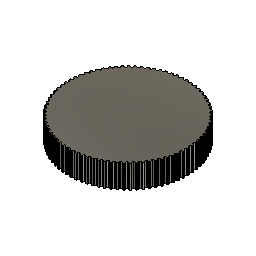
gear_81z (Autodesk Fusion 360 design; units mm, degrees)
Autodesk Fusion 360 part; units mm, degrees
sketch "Sketch1" plane through (0, 0, 0) normal (0, 0, 1) x (1, 0, 0) in component "gt2 pulley"
  circle A0 centre (0, 0) radius 25.7831 construction
  circle A1 centre (0, 0) radius 24.7791 construction
  line L0 (0, 0) -> (0, 25.7831) construction
  line L1 (0, 0) -> (0.9997, 25.7637) construction
  line L2 (0, 0) -> (1.4048, 25.7448) construction
  circle A2 centre (0, 0) radius 25.5291 construction
  arc A3 (0.3959, 25.3927) -> (0.4727, 25.0954) centre (1.391, 25.4912) ccw
  circle A4 centre (0, 0) radius 25.3791 construction
  arc A5 (0.248, 25.5279) -> (0, 25.5291) centre (0, 0) ccw
  arc A6 (0.3959, 25.3927) -> (0.248, 25.5279) centre (0.2466, 25.3779) ccw
  arc A7 (0.4727, 25.0954) -> (0.9608, 24.7605) centre (0.9823, 25.315) ccw
  arc A8 (0, 25.5291) -> (-0.248, 25.5279) centre (0, 0) ccw
  arc A9 (-0.248, 25.5279) -> (-0.3959, 25.3927) centre (-0.2466, 25.3779) ccw
  arc A10 (-0.4727, 25.0954) -> (-0.3959, 25.3927) centre (-1.391, 25.4912) ccw
  arc A11 (-0.9607, 24.7605) -> (-0.4727, 25.0954) centre (-0.9823, 25.315) ccw
  arc A12 (0.9608, 24.7605) -> (-0.9608, 24.7605) centre (0, 0) ccw
  point P0 (1.391, 25.4912)
  point P1 (0, 25.5291)
  dimension "d18" = 51.5662
  dimension "d19" = 2.222
  dimension "d22" = 1.004
  dimension "d24" = 0.75
  dimension "d26" = 1
  dimension "d27" = 0.15
  dimension "d28" = 0.15
  dimension "d47" = 0.555
  dimension "d52" = 3.812
  constraint coincident A0.centre A1.centre
  constraint coincident A0 L0.end
  constraint vertical L0
  constraint coincident A0 L1.end
  constraint coincident A0 L2.end
  constraint concentric A1 A2
  constraint coincident A1 A7.end
  constraint coincident L1 A7.end
  constraint coincident A2 P0
  constraint coincident L2 P0
  constraint coincident P0 A3.centre
  constraint coincident A2 P1
  constraint coincident L0 P1
  constraint concentric A2 A4
  constraint coincident P1 A5.end
  constraint coincident A4 A6.centre
  constraint coincident A3.start A6.start
  constraint tangent A3 A6
  constraint tangent A3 A7
  constraint symmetric L0 A7.end A12.end
  constraint symmetric L0 A3.start A9.end
  constraint symmetric L0 A3.end A10.start
  constraint symmetric L0 A3 A10
  constraint symmetric L0 A5.start A8.end
  constraint symmetric L0 P1 A5.end
  constraint symmetric L0 A5 A8
  constraint symmetric L0 A6 A9
  constraint symmetric L0 A7 A11
  constraint coincident A1 A11.start
  constraint tangent A1 A7
  constraint coincident L1 A7.centre
  measures "d18" diameter of A0
  measures "d19" angle of L0 L1
  measures "d22" distance of A0 A1
  measures "d24" distance of A1 A2
  measures "d26" radius of A3
  measures "d27" distance of A2 A4
  measures "d28" radius of A6
  measures "d47" radius of A7
extrude "Extrude1" add sketch "Sketch1" along normal blind 10 makes body 1
pattern_circular "C-Pattern1" count 81 over 360 about axis through (0, 0, 1.75) along (0, 0, 1) of bodies 1 makes body 2 at (-1.1742, 24.7513, 3.3333) makes body 3 at (-4.3553, 24.3933, 6.6667) makes body 4 at (-4.9846, 24.2726, 3.3333) makes body 5 at (-8.0723, 23.4274, 6.6667) makes body 6 at (-8.6753, 23.2108, 3.3333) makes body 7 at (-11.7836, 21.798, 6.6667) makes body 8 at (-12.1576, 21.5916, 3.3333) makes body 9 at (-14.8398, 19.844, 6.6667) makes body 10 at (-16.4929, 18.4929, 6.6667) makes body 11 at (-17.7278, 17.3126, 6.6667) makes body 12 at (-18.1695, 16.8485, 3.3333) makes body 13 at (-19.9394, 14.7113, 6.6667) makes body 14 at (-21.0195, 13.1219, 6.6667) makes body 15 at (-22.1673, 11.0732, 6.6667) makes body 16 at (-22.7946, 9.7164, 6.6667) makes body 17 at (-23.1921, 8.7253, 3.3333) makes body 18 at (-24.0222, 6.0775, 6.6667) makes body 19 at (-24.5213, 3.5649, 6.6667) makes body 20 at (-24.5791, 3.1417, 3.3333) makes body 21 at (-24.7487, 1.2275, 3.3333) makes body 22 at (-24.6825, -2.1862, 6.6667) makes body 23 at (-24.4388, -4.0923, 6.6667) makes body 24 at (-24.3647, -4.513, 3.3333) makes body 25 at (-23.513, -7.8194, 6.6667) makes body 26 at (-23.1543, -8.8251, 6.6667) makes body 27 at (-22.3086, -10.7856, 6.6667) makes body 28 at (-21.8233, -11.7367, 3.3333) makes body 29 at (-20.8481, -13.3925, 3.3333) makes body 30 at (-19.7476, -14.9678, 3.3333) makes body 31 at (-18.5284, -16.4531, 3.3333) makes body 32 at (-16.0908, -18.8439, 6.6667) makes body 33 at (-14.5821, -20.0341, 6.6667) makes body 34 at (-14.2346, -20.2825, 3.3333) makes body 35 at (-11.5009, -21.9484, 6.6667) makes body 36 at (-9.5689, -22.857, 6.6667) makes body 37 at (-7.7689, -23.5297, 6.6667) makes body 38 at (-5.9221, -24.061, 6.6667) makes body 39 at (-4.6705, -24.335, 6.6667) makes body 40 at (-2.3458, -24.6678, 6.6667) makes body 41 at (-1.7072, -24.7202, 3.3333) makes body 42 at (1.7071, -24.7202, 6.6667) makes body 43 at (2.133, -24.6871, 3.3333) makes body 44 at (5.5064, -24.1596, 6.6667) makes body 45 at (6.7478, -23.8426, 6.6667) makes body 46 at (8.3745, -23.3211, 6.6667) makes body 47 at (10.9295, -22.2385, 6.6667) makes body 48 at (11.3113, -22.0467, 3.3333) makes body 49 at (12.9857, -21.1039, 3.3333) makes body 50 at (14.5821, -20.0342, 3.3333) makes body 51 at (16.0907, -18.8439, 3.3333) makes body 52 at (18.5283, -16.4532, 6.6667) makes body 53 at (18.8092, -16.1313, 3.3333) makes body 54 at (20.4949, -13.9271, 6.6667) makes body 55 at (21.5125, -12.297, 6.6667) makes body 56 at (22.4007, -10.593, 6.6667) makes body 57 at (23.3747, -8.2237, 6.6667) makes body 58 at (23.9416, -6.3876, 6.6667) makes body 59 at (24.3646, -4.5131, 6.6667) makes body 60 at (24.4388, -4.0924, 3.3333) makes body 61 at (24.6825, -2.1862, 3.3333) makes body 62 at (24.7777, -0.267, 3.3333) makes body 63 at (24.7238, 1.6539, 3.3333) makes body 64 at (24.3839, 4.4079, 6.6667) makes body 65 at (23.7985, 6.9018, 6.6667) makes body 66 at (23.676, 7.311, 3.3333) makes body 67 at (23.0382, 9.1238, 3.3333) makes body 68 at (21.5654, 12.2041, 6.6667) makes body 69 at (20.5548, 13.8385, 6.6667) makes body 70 at (19.4206, 15.3897, 6.6667) makes body 71 at (18.1696, 16.8484, 6.6667) makes body 72 at (17.8764, 17.1592, 3.3333) makes body 73 at (15.348, 19.4536, 6.6667) makes body 74 at (14.4956, 20.0968, 6.6667) makes body 75 at (13.4374, 20.8192, 3.3333) makes body 76 at (11.7837, 21.7979, 3.3333) makes body 77 at (10.0591, 22.6455, 3.3333) makes body 78 at (6.8507, 23.8133, 6.6667) makes body 79 at (4.9847, 24.2725, 6.6667) makes body 80 at (4.5655, 24.3549, 3.3333) makes body 81 at (1.1743, 24.7513, 6.6667)
sketch "Sketch2" plane through (0, 0, 10) normal (0, 0, 1) x (-1, 0, 0)
  arc A0 (-11.75, -22.5141) -> (-11.6785, -22.7013) centre (-11.6099, -22.5679) ccw
  arc A1 (-11.6785, -22.7013) -> (-11.2353, -22.9239) centre (0, 0) ccw
  arc A2 (-11.2353, -22.9239) -> (-11.0425, -22.8694) centre (-11.1692, -22.7892) ccw
  arc A3 (-10.8404, -22.6382) -> (-11.0425, -22.8694) centre (-10.1974, -23.404) ccw
  arc A4 (-10.2539, -22.5579) -> (-10.8404, -22.6382) centre (-10.4835, -23.0632) ccw
  arc A5 (-11.9711, -21.6955) -> (-10.2539, -22.5579) centre (0, 0) ccw
  arc A6 (-11.6852, -22.2139) -> (-11.9711, -21.6955) centre (-12.2392, -22.1815) ccw
  arc A7 (-11.75, -22.5141) -> (-11.6852, -22.2139) centre (-12.6835, -22.1555) ccw
  circle A8 centre (0, 0) radius 24.7791
  constraint concentric A1 A8
extrude "Extrude2" add sketch "Sketch2" against normal blind 10 contours A5 A8 bodies 1 2 3 4 5 6 7 8 9 10 11 12 13 14 15 16 17 18 19 20 21 22 23 24 25 26 27 28 29 30 31 32 33 34 35 36 37 38 39 40 41 42 43 44 45 46 47 48 49 50 51 52 53 54 55 56 57 58 59 60 61 62 63 64 65 66 67 68 69 70 71 72 73 74 75 76 77 78 79 80 81
extrude "Extrude4" [suppressed] in component "gt2 pulley"
pattern_circular "C-Pattern7" [suppressed] in component "gt2 pulley"
extrude "Extrude3" [suppressed] in component "gt2 pulley"
pattern_circular "C-Pattern6" [suppressed] in component "gt2 pulley"
extrude "Extrude2'" [suppressed] in component "gt2 pulley"
pattern_circular "C-Pattern5" [suppressed] in component "gt2 pulley"
extrude "Extrude1'" [suppressed] in component "gt2 pulley"
pattern_circular "C-Pattern4" [suppressed] in component "gt2 pulley"
pattern_circular "C-Pattern3" [suppressed] in component "gt2 pulley"
pattern_circular "C-Pattern2" [suppressed] in component "gt2 pulley"
pattern_circular "C-Pattern1'" [suppressed] in component "gt2 pulley"
copy_body "Body->Comp1" [suppressed] in component "Component"
copy_body "Body->Comp2" [suppressed] in component "Component'"
copy_body "Body->Comp3" [suppressed] in component "Component''"
copy_body "Body->Comp4" [suppressed] in component "Component'''"
copy_body "Body->Comp5" [suppressed] in component "Component''''"
copy_body "Body->Comp6" [suppressed] in component "Component'''''"
copy_body "Body->Comp7" [suppressed] in component "Component''''''"
copy_body "Body->Comp8" [suppressed] in component "Component'''''''"
copy_body "Body->Comp9" [suppressed] in component "Component''''''''"
copy_body "Body->Comp10" [suppressed] in component "Component'''''''''"
copy_body "Body->Comp11" [suppressed] in component "Component''''''''''"
copy_body "Body->Comp12" [suppressed] in component "Component'''''''''''"
copy_body "Body->Comp13" [suppressed] in component "Component''''''''''''"
copy_body "Body->Comp14" [suppressed] in component "Component'''''''''''''"
copy_body "Body->Comp15" [suppressed] in component "Component''''''''''''''"
copy_body "Body->Comp16" [suppressed] in component "Component'''''''''''''''"
copy_body "Body->Comp17" [suppressed] in component "Component''''''''''''''''"
copy_body "Body->Comp18" [suppressed] in component "Component'''''''''''''''''"
copy_body "Body->Comp19" [suppressed] in component "Component''''''''''''''''''"
copy_body "Body->Comp20" [suppressed] in component "Component'''''''''''''''''''"
component "gt2 pulley" placed x (1, 0, 0) y (0, 1, 0) z (0, 0, 1) at (0, 0, 0)
equation "NumTeeth = 81" comment "min 20"
equation "ToothPitch = 2 mm"
equation "PullyDia = NumTeeth * ToothPitch / PI"
equation "ToothAng = ( ( 360 / NumTeeth ) * 1 deg )"
equation "TransOffsetAngle = ToothAng * 0.2"
equation "Sholulder_Radius = 0.15 mm"
equation "Root_Radius = 0.555 mm"
equation "TransRadius = 1 mm"
equation "ToolHeight = 0.75 mm"
equation "PLD = 0.254 mm"
equation "d18 = PullyDia"
equation "d19 = ToothAng / 2"
equation "d22 = PLD + ToolHeight"
equation "d24 = ToolHeight"
equation "d26 = TransRadius"
equation "d27 = Sholulder_Radius"
equation "d31 = NumTeeth"
equation "d33 = NumTeeth"
equation "d35 = NumTeeth"
equation "d37 = NumTeeth"
equation "d41 = NumTeeth"
equation "d45 = NumTeeth"
equation "d47 = Root_Radius"
equation "d50 = NumTeeth"
